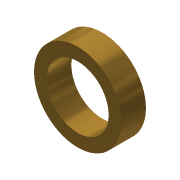
# Autodesk Inventor part: Module Live Axle Thrust Bearing Bushing
Saved by Autodesk Inventor 2014 SP1 (Build 180222100, 222)
## iProperties
Created: 2014-05-04
Part Number: Module Live Axle Thrust Bearing Bushing
Material: Brass, Soft Yellow
Document SubType Name: Modeling
Designer: Rauhul Varma
Mass: 1.90779 g
Surface Area: 3.69623 cm^2
Volume: 0.225241 cm^3
Density: 8.47 g/cm^3
Appearance: Brass - Satin
Author: Rauhul Varma
Autodesk Inventor part; units mm, degrees
ref_plane "YZ Plane" through (0, 0, 0) normal (1, 0, 0) x (0, 1, 0)
ref_plane "XZ Plane" through (0, 0, 0) normal (0, 1, 0) x (-1, 0, 0)
ref_plane "XY Plane" through (0, 0, 0) normal (0, 0, 1) x (1, 0, 0)
sketch "Sketch1" plane through (0, 0, 0) normal (0, 0, 1) x (1, 0, 0)
  circle A0 centre (0, 0) radius 4.5
  circle A1 centre (0, 0) radius 6.35
  dimension "d0" = 9
  dimension "d1" = 12.7
  constraints: 2 centre point, 2 coincident
  measures "d0" diameter of A0
  measures "d1" diameter of A1
extrude "Extrusion1" add sketch "Sketch1" along normal blind 3.5719
body "Solid1"
